Autodesk Inventor part; units mm, degrees
(part 2 of 2)
sketch "スケッチ13" plane through (0, 0, -5) normal (0, 0, -1) x (-1, 0, 0)
  arc A0 (74.152214, 49.824752) -> (76.907606, 48.647957) centre (77.811872, 54.579424) ccw
  arc A1 (74.152214, 49.824752) -> (72.542276, 49.029257) centre (73.542271, 49.032306) ccw
  arc A2 (70.331118, 43.4429) -> (72.542276, 49.029257) centre (64.442314, 49.004554) ccw
  arc A3 (70.331118, 43.4429) -> (70.457765, 41.956551) centre (71.058131, 42.756277) ccw
  line L0 (70.457765, 41.956551) -> (77.631528, 36.571106)
  arc A4 (77.631528, 36.571106) -> (79.072459, 36.829123) centre (78.231893, 37.370832) ccw
  arc A5 (80.094406, 38.031727) -> (79.072459, 36.829123) centre (84.115857, 33.578871) ccw
  arc A6 (80.094406, 38.031727) -> (80.381942, 39.061377) centre (79.424164, 38.77387) ccw
  line L1 (80.381942, 39.061377) -> (77.714673, 47.946886)
  arc A7 (77.714673, 47.946886) -> (76.907606, 48.647957) centre (76.756895, 47.659379) ccw
  arc A8 (137.500173, 2.708082) -> (138.19969, 1.899667) centre (138.489039, 2.856891) ccw
  arc A9 (142.031716, -1.608501) -> (138.19969, 1.899667) centre (136.463592, -3.843674) ccw
  arc A10 (142.031716, -1.608501) -> (143.581885, -2.018871) centre (142.959736, -1.235972) ccw
  line L2 (143.581885, -2.018871) -> (146.594315, 0.375026)
  arc A11 (146.594315, 0.375026) -> (146.254963, 2.117105) centre (145.972167, 1.157925) ccw
  arc A12 (142.242708, 6.02639) -> (146.254963, 2.117105) centre (147.951739, 7.872185) ccw
  arc A13 (142.242708, 6.02639) -> (141.421042, 6.710292) centre (141.291203, 5.718757) ccw
  line L3 (141.421042, 6.710292) -> (138.123227, 7.142135)
  arc A14 (138.123227, 7.142135) -> (137.004522, 6.001791) centre (137.993388, 6.1506) ccw
  line L4 (137.004522, 6.001791) -> (137.500173, 2.708082)
  arc A15 (136.03468, 16.286601) -> (138.023268, 18.525143) centre (132.685182, 21.264639) ccw
  arc A16 (136.03468, 16.286601) -> (135.604064, 15.308119) centre (136.59293, 15.456928) ccw
  line L5 (135.604064, 15.308119) -> (136.075602, 12.174654)
  arc A17 (136.075602, 12.174654) -> (136.934628, 11.331928) centre (137.064468, 12.323463) ccw
  line L6 (136.934628, 11.331928) -> (141.9404, 10.676432)
  arc A18 (141.9404, 10.676432) -> (142.910454, 11.125713) centre (142.07024, 11.667967) ccw
  arc A19 (145.546046, 13.368787) -> (142.910454, 11.125713) centre (147.951739, 7.872185) ccw
  arc A20 (145.546046, 13.368787) -> (145.664062, 15.139683) centre (145.145097, 14.284888) ccw
  line L7 (145.664062, 15.139683) -> (139.431914, 18.923356)
  arc A21 (139.431914, 18.923356) -> (138.023268, 18.525143) centre (138.912949, 18.068561) ccw
  arc A22 (100.355268, 41.394209) -> (100.058689, 42.827701) centre (99.539724, 41.972905) ccw
  line L8 (100.058689, 42.827701) -> (84.558604, 52.238141)
  arc A23 (84.558604, 52.238141) -> (83.149958, 51.839928) centre (84.039639, 51.383346) ccw
  arc A24 (81.833323, 50.126568) -> (83.149958, 51.839928) centre (77.811872, 54.579424) ccw
  arc A25 (81.833323, 50.126568) -> (81.545787, 49.096917) centre (82.503565, 49.384425) ccw
  line L9 (81.545787, 49.096917) -> (84.213055, 40.211408)
  arc A26 (84.213055, 40.211408) -> (85.020123, 39.510338) centre (85.170834, 40.498916) ccw
  arc A27 (88.908264, 37.188973) -> (85.020123, 39.510338) centre (84.115857, 33.578871) ccw
  arc A28 (88.908264, 37.188973) -> (89.908309, 36.81113) centre (89.706998, 37.790657) ccw
  line L10 (89.908309, 36.81113) -> (98.650829, 38.607882)
  arc A29 (98.650829, 38.607882) -> (99.420805, 39.349498) centre (98.449518, 39.587409) ccw
  arc A30 (100.355268, 41.394209) -> (99.420805, 39.349498) centre (105.248527, 37.922031) ccw
  arc A31 (70.160292, 54.741689) -> (71.858452, 55.325612) centre (70.866216, 55.449977) ccw
  arc A32 (72.918613, 58.051601) -> (71.858452, 55.325612) centre (77.811872, 54.579424) ccw
  arc A33 (72.918613, 58.051601) -> (72.622035, 59.485093) centre (72.10307, 58.630298) ccw
  line L11 (72.622035, 59.485093) -> (69.229438, 61.544813)
  arc A34 (69.229438, 61.544813) -> (67.802662, 61.109398) centre (68.710473, 60.690017) ccw
  arc A35 (66.414464, 59.026602) -> (67.802662, 61.109398) centre (60.449397, 64.50638) ccw
  arc A36 (66.414464, 59.026602) -> (66.550527, 57.55036) centre (67.150892, 58.350086) ccw
  line L12 (66.550527, 57.55036) -> (69.305274, 55.482332)
  arc A37 (70.160292, 54.741689) -> (69.305274, 55.482332) centre (64.442314, 49.004554) ccw
  arc A38 (127.791923, 24.736817) -> (126.690727, 21.522538) centre (132.685182, 21.264639) ccw
  arc A39 (127.791923, 24.736817) -> (127.495344, 26.170308) centre (126.976379, 25.315513) ccw
  line L13 (127.495344, 26.170308) -> (111.995259, 35.580749)
  arc A40 (111.995259, 35.580749) -> (110.586613, 35.182536) centre (111.476294, 34.725953) ccw
  arc A41 (109.14609, 33.360343) -> (110.586613, 35.182536) centre (105.248527, 37.922031) ccw
  arc A42 (109.14609, 33.360343) -> (108.830366, 32.338983) centre (109.795684, 32.600062) ccw
  line L14 (108.830366, 32.338983) -> (112.38569, 19.19344)
  arc A43 (112.38569, 19.19344) -> (113.173186, 18.470456) centre (113.351007, 19.454519) ccw
  arc A44 (116.098395, 17.045236) -> (113.173186, 18.470456) centre (112.106259, 12.566079) ccw
  arc A45 (116.098395, 17.045236) -> (117.15309, 16.870668) centre (116.763751, 17.791763) ccw
  line L15 (117.15309, 16.870668) -> (126.080991, 20.644427)
  arc A46 (126.080991, 20.644427) -> (126.690727, 21.522538) centre (125.691651, 21.565521) ccw
  line L16 (123.324226, 13.114183) -> (130.745103, 12.142434)
  arc A47 (130.745103, 12.142434) -> (131.863809, 13.282778) centre (130.874943, 13.133969) ccw
  line L17 (131.863809, 13.282778) -> (131.6486, 14.712884)
  arc A48 (131.6486, 14.712884) -> (130.949084, 15.521298) centre (130.659734, 14.564075) ccw
  arc A49 (128.693046, 16.785482) -> (130.949084, 15.521298) centre (132.685182, 21.264639) ccw
  arc A50 (128.693046, 16.785482) -> (127.63835, 16.96005) centre (128.02769, 16.038956) ccw
  line L18 (127.63835, 16.96005) -> (123.064726, 15.026812)
  arc A51 (123.064726, 15.026812) -> (123.324226, 13.114183) centre (123.454066, 14.105718) ccw
  arc A52 (88.644656, 29.643139) -> (88.79909, 28.187458) centre (89.399456, 28.987184) ccw
  line L19 (88.79909, 28.187458) -> (105.621929, 15.558314)
  arc A53 (105.621929, 15.558314) -> (107.062861, 15.816331) centre (106.222295, 16.35804) ccw
  arc A54 (108.208695, 17.127767) -> (107.062861, 15.816331) centre (112.106259, 12.566079) ccw
  arc A55 (108.208695, 17.127767) -> (108.524419, 18.149127) centre (107.559102, 17.888049) ccw
  line L20 (108.524419, 18.149127) -> (104.969096, 31.29467)
  arc A56 (104.969096, 31.29467) -> (104.181599, 32.017655) centre (104.003778, 31.033592) ccw
  arc A57 (100.45612, 34.311929) -> (104.181599, 32.017655) centre (105.248527, 37.922031) ccw
  arc A58 (100.45612, 34.311929) -> (99.456074, 34.689773) centre (99.657386, 33.710245) ccw
  line L21 (99.456074, 34.689773) -> (90.713554, 32.89302)
  arc A59 (90.713554, 32.89302) -> (89.943579, 32.151404) centre (90.914866, 31.913493) ccw
  arc A60 (88.644656, 29.643139) -> (89.943579, 32.151404) centre (84.115857, 33.578871) ccw
  arc A61 (133.114093, 1.134364) -> (133.54471, 2.112846) centre (132.555844, 1.964037) ccw
  line L22 (133.54471, 2.112846) -> (132.792729, 7.109914)
  arc A62 (132.792729, 7.109914) -> (131.933702, 7.95264) centre (131.803863, 6.961105) ccw
  line L23 (131.933702, 7.95264) -> (118.117598, 9.761832)
  arc A63 (118.117598, 9.761832) -> (117.147544, 9.312551) centre (117.987758, 8.770297) ccw
  arc A64 (116.635058, 8.630348) -> (117.147544, 9.312551) centre (112.106259, 12.566079) ccw
  arc A65 (116.635058, 8.630348) -> (116.789492, 7.174667) centre (117.389857, 7.974392) ccw
  line L24 (116.789492, 7.174667) -> (129.297772, -2.215477)
  arc A66 (129.297772, -2.215477) -> (130.83606, -1.762597) centre (129.898137, -1.415751) ccw
  arc A67 (133.114093, 1.134364) -> (130.83606, -1.762597) centre (136.463592, -3.843674) ccw
  circle A68 centre (105.248527, 37.922031) radius 3
  circle A69 centre (132.685182, 21.264639) radius 3
  circle A70 centre (77.811872, 54.579424) radius 3
  circle A71 centre (112.106259, 12.566079) radius 3
  circle A72 centre (84.115857, 33.578871) radius 3
  circle A73 centre (136.463592, -3.843674) radius 3
  circle A74 centre (147.951739, 7.872185) radius 3
  line L25 (46.496021, 71.105048) -> (58.588264, 62.02723)
  arc A75 (58.588264, 62.02723) -> (62.310529, 66.98553) centre (60.449397, 64.50638) ccw
  line L26 (62.310529, 66.98553) -> (56.416161, 71.410515)
  line L27 (56.416161, 71.410515) -> (60.233181, 71.528052)
  arc A76 (64.095126, 70.511318) -> (60.233181, 71.528052) centre (60.449397, 64.50638) ccw
  line L28 (64.095126, 70.511318) -> (136.058454, 26.82081)
  arc A77 (136.850058, 26.255011) -> (136.058454, 26.82081) centre (132.685182, 21.264639) ccw
  line L29 (136.850058, 26.255011) -> (152.436991, 13.246431)
  arc A78 (153.239213, 3.284961) -> (152.436991, 13.246431) centre (147.951739, 7.872185) ccw
  line L30 (153.239213, 3.284961) -> (142.506418, -9.086216)
  arc A79 (131.660668, -10.24148) -> (142.506418, -9.086216) centre (136.463592, -3.843674) ccw
  line L31 (131.660668, -10.24148) -> (40.231602, 58.395617)
  arc A80 (37.546552, 65.319255) -> (40.231602, 58.395617) centre (44.44917, 64.013691) ccw
  line L32 (37.546552, 65.319255) -> (62.581181, 46.525404)
  arc A81 (62.581181, 46.525404) -> (66.303447, 51.483704) centre (64.442314, 49.004554) ccw
  line L33 (66.303447, 51.483704) -> (41.268818, 70.277554)
  arc A82 (44.232954, 71.035362) -> (41.268818, 70.277554) centre (44.44917, 64.013691) ccw
  line L34 (44.232954, 71.035362) -> (46.496021, 71.105048)
  circle A83 centre (147.951739, 7.872185) radius 7
  point P0 (0, 0)
  point P1 (146.087496, 14.619377)
  point P2 (141.559999, 10.726245)
  point P3 (141.040641, 6.760105)
  point P4 (146.949096, 0.944364)
  dimension "d69" = 4
  constraints: 1 centre point, 1 coincident
  measures "d69" radial gap between concentric circles of A74 A83
extrude "押し出し11" add sketch "スケッチ13" against normal blind 5 contours L3 A13 A12 A11 A83 | A83 A20 A19 A18 L6
fillet "フィレット2" radius 1 2 edges at (-146.9491, 0.9444, -3) (-146.0875, 14.6194, -3)
fillet "フィレット3" radius 1 2 edges at (-141.0406, 6.7601, -3) (-141.56, 10.7262, -3)
sketch "スケッチ14" plane through (0, 0, -5) normal (0, 0, -1) x (-1, 0, 0)
  arc A0 (74.152214, 49.824752) -> (76.907606, 48.647957) centre (77.811872, 54.579424) ccw
  arc A1 (74.152214, 49.824752) -> (72.542276, 49.029257) centre (73.542271, 49.032306) ccw
  arc A2 (70.331118, 43.4429) -> (72.542276, 49.029257) centre (64.442314, 49.004554) ccw
  arc A3 (70.331118, 43.4429) -> (70.457765, 41.956551) centre (71.058131, 42.756277) ccw
  line L0 (70.457765, 41.956551) -> (77.631528, 36.571106)
  arc A4 (77.631528, 36.571106) -> (79.072459, 36.829123) centre (78.231893, 37.370832) ccw
  arc A5 (80.094406, 38.031727) -> (79.072459, 36.829123) centre (84.115857, 33.578871) ccw
  arc A6 (80.094406, 38.031727) -> (80.381942, 39.061377) centre (79.424164, 38.77387) ccw
  line L1 (80.381942, 39.061377) -> (77.714673, 47.946886)
  arc A7 (77.714673, 47.946886) -> (76.907606, 48.647957) centre (76.756895, 47.659379) ccw
  arc A8 (137.500173, 2.708082) -> (138.19969, 1.899667) centre (138.489039, 2.856891) ccw
  arc A9 (142.031716, -1.608501) -> (138.19969, 1.899667) centre (136.463592, -3.843674) ccw
  arc A10 (142.031716, -1.608501) -> (143.581885, -2.018871) centre (142.959736, -1.235972) ccw
  line L2 (143.581885, -2.018871) -> (145.665299, -0.363238)
  arc A11 (145.665299, -0.363238) -> (145.406724, 1.351227) centre (145.043151, 0.419661) ccw
  arc A12 (141.176668, 6.111957) -> (145.406724, 1.351227) centre (147.951739, 7.872185) ccw
  arc A13 (141.176668, 6.111957) -> (140.33864, 6.852031) centre (140.2088, 5.860496) ccw
  line L3 (140.33864, 6.852031) -> (138.123227, 7.142135)
  arc A14 (138.123227, 7.142135) -> (137.004522, 6.001791) centre (137.993388, 6.1506) ccw
  line L4 (137.004522, 6.001791) -> (137.500173, 2.708082)
  arc A15 (136.03468, 16.286601) -> (138.023268, 18.525143) centre (132.685182, 21.264639) ccw
  arc A16 (136.03468, 16.286601) -> (135.604064, 15.308119) centre (136.59293, 15.456928) ccw
  line L5 (135.604064, 15.308119) -> (136.075602, 12.174654)
  arc A17 (136.075602, 12.174654) -> (136.934628, 11.331928) centre (137.064468, 12.323463) ccw
  line L6 (136.934628, 11.331928) -> (140.857998, 10.818171)
  arc A18 (140.857998, 10.818171) -> (141.858325, 11.317516) centre (140.987838, 11.809706) ccw
  arc A19 (144.608388, 14.022144) -> (141.858325, 11.317516) centre (147.951739, 7.872185) ccw
  arc A20 (144.608388, 14.022144) -> (144.649731, 15.755505) centre (144.130766, 14.90071) ccw
  line L7 (144.649731, 15.755505) -> (139.431914, 18.923356)
  arc A21 (139.431914, 18.923356) -> (138.023268, 18.525143) centre (138.912949, 18.068561) ccw
  arc A22 (100.355268, 41.394209) -> (100.058689, 42.827701) centre (99.539724, 41.972905) ccw
  line L8 (100.058689, 42.827701) -> (84.558604, 52.238141)
  arc A23 (84.558604, 52.238141) -> (83.149958, 51.839928) centre (84.039639, 51.383346) ccw
  arc A24 (81.833323, 50.126568) -> (83.149958, 51.839928) centre (77.811872, 54.579424) ccw
  arc A25 (81.833323, 50.126568) -> (81.545787, 49.096917) centre (82.503565, 49.384425) ccw
  line L9 (81.545787, 49.096917) -> (84.213055, 40.211408)
  arc A26 (84.213055, 40.211408) -> (85.020123, 39.510338) centre (85.170834, 40.498916) ccw
  arc A27 (88.908264, 37.188973) -> (85.020123, 39.510338) centre (84.115857, 33.578871) ccw
  arc A28 (88.908264, 37.188973) -> (89.908309, 36.81113) centre (89.706998, 37.790657) ccw
  line L10 (89.908309, 36.81113) -> (98.650829, 38.607882)
  arc A29 (98.650829, 38.607882) -> (99.420805, 39.349498) centre (98.449518, 39.587409) ccw
  arc A30 (100.355268, 41.394209) -> (99.420805, 39.349498) centre (105.248527, 37.922031) ccw
  arc A31 (70.160292, 54.741689) -> (71.858452, 55.325612) centre (70.866216, 55.449977) ccw
  arc A32 (72.918613, 58.051601) -> (71.858452, 55.325612) centre (77.811872, 54.579424) ccw
  arc A33 (72.918613, 58.051601) -> (72.622035, 59.485093) centre (72.10307, 58.630298) ccw
  line L11 (72.622035, 59.485093) -> (69.229438, 61.544813)
  arc A34 (69.229438, 61.544813) -> (67.802662, 61.109398) centre (68.710473, 60.690017) ccw
  arc A35 (66.414464, 59.026602) -> (67.802662, 61.109398) centre (60.449397, 64.50638) ccw
  arc A36 (66.414464, 59.026602) -> (66.550527, 57.55036) centre (67.150892, 58.350086) ccw
  line L12 (66.550527, 57.55036) -> (69.305274, 55.482332)
  arc A37 (70.160292, 54.741689) -> (69.305274, 55.482332) centre (64.442314, 49.004554) ccw
  arc A38 (127.791923, 24.736817) -> (126.690727, 21.522538) centre (132.685182, 21.264639) ccw
  arc A39 (127.791923, 24.736817) -> (127.495344, 26.170308) centre (126.976379, 25.315513) ccw
  line L13 (127.495344, 26.170308) -> (111.995259, 35.580749)
  arc A40 (111.995259, 35.580749) -> (110.586613, 35.182536) centre (111.476294, 34.725953) ccw
  arc A41 (109.14609, 33.360343) -> (110.586613, 35.182536) centre (105.248527, 37.922031) ccw
  arc A42 (109.14609, 33.360343) -> (108.830366, 32.338983) centre (109.795684, 32.600062) ccw
  line L14 (108.830366, 32.338983) -> (112.38569, 19.19344)
  arc A43 (112.38569, 19.19344) -> (113.173186, 18.470456) centre (113.351007, 19.454519) ccw
  arc A44 (116.098395, 17.045236) -> (113.173186, 18.470456) centre (112.106259, 12.566079) ccw
  arc A45 (116.098395, 17.045236) -> (117.15309, 16.870668) centre (116.763751, 17.791763) ccw
  line L15 (117.15309, 16.870668) -> (126.080991, 20.644427)
  arc A46 (126.080991, 20.644427) -> (126.690727, 21.522538) centre (125.691651, 21.565521) ccw
  line L16 (123.324226, 13.114183) -> (130.745103, 12.142434)
  arc A47 (130.745103, 12.142434) -> (131.863809, 13.282778) centre (130.874943, 13.133969) ccw
  line L17 (131.863809, 13.282778) -> (131.6486, 14.712884)
  arc A48 (131.6486, 14.712884) -> (130.949084, 15.521298) centre (130.659734, 14.564075) ccw
  arc A49 (128.693046, 16.785482) -> (130.949084, 15.521298) centre (132.685182, 21.264639) ccw
  arc A50 (128.693046, 16.785482) -> (127.63835, 16.96005) centre (128.02769, 16.038956) ccw
  line L18 (127.63835, 16.96005) -> (123.064726, 15.026812)
  arc A51 (123.064726, 15.026812) -> (123.324226, 13.114183) centre (123.454066, 14.105718) ccw
  arc A52 (88.644656, 29.643139) -> (88.79909, 28.187458) centre (89.399456, 28.987184) ccw
  line L19 (88.79909, 28.187458) -> (105.621929, 15.558314)
  arc A53 (105.621929, 15.558314) -> (107.062861, 15.816331) centre (106.222295, 16.35804) ccw
  arc A54 (108.208695, 17.127767) -> (107.062861, 15.816331) centre (112.106259, 12.566079) ccw
  arc A55 (108.208695, 17.127767) -> (108.524419, 18.149127) centre (107.559102, 17.888049) ccw
  line L20 (108.524419, 18.149127) -> (104.969096, 31.29467)
  arc A56 (104.969096, 31.29467) -> (104.181599, 32.017655) centre (104.003778, 31.033592) ccw
  arc A57 (100.45612, 34.311929) -> (104.181599, 32.017655) centre (105.248527, 37.922031) ccw
  arc A58 (100.45612, 34.311929) -> (99.456074, 34.689773) centre (99.657386, 33.710245) ccw
  line L21 (99.456074, 34.689773) -> (90.713554, 32.89302)
  arc A59 (90.713554, 32.89302) -> (89.943579, 32.151404) centre (90.914866, 31.913493) ccw
  arc A60 (88.644656, 29.643139) -> (89.943579, 32.151404) centre (84.115857, 33.578871) ccw
  arc A61 (133.114093, 1.134364) -> (133.54471, 2.112846) centre (132.555844, 1.964037) ccw
  line L22 (133.54471, 2.112846) -> (132.792729, 7.109914)
  arc A62 (132.792729, 7.109914) -> (131.933702, 7.95264) centre (131.803863, 6.961105) ccw
  line L23 (131.933702, 7.95264) -> (118.117598, 9.761832)
  arc A63 (118.117598, 9.761832) -> (117.147544, 9.312551) centre (117.987758, 8.770297) ccw
  arc A64 (116.635058, 8.630348) -> (117.147544, 9.312551) centre (112.106259, 12.566079) ccw
  arc A65 (116.635058, 8.630348) -> (116.789492, 7.174667) centre (117.389857, 7.974392) ccw
  line L24 (116.789492, 7.174667) -> (129.297772, -2.215477)
  arc A66 (129.297772, -2.215477) -> (130.83606, -1.762597) centre (129.898137, -1.415751) ccw
  arc A67 (133.114093, 1.134364) -> (130.83606, -1.762597) centre (136.463592, -3.843674) ccw
  circle A68 centre (105.248527, 37.922031) radius 3
  circle A69 centre (132.685182, 21.264639) radius 3
  circle A70 centre (77.811872, 54.579424) radius 3
  circle A71 centre (112.106259, 12.566079) radius 3
  circle A72 centre (84.115857, 33.578871) radius 3
  circle A73 centre (136.463592, -3.843674) radius 3
  circle A74 centre (147.951739, 7.872185) radius 3
  line L25 (46.496021, 71.105048) -> (58.588264, 62.02723)
  arc A75 (58.588264, 62.02723) -> (62.310529, 66.98553) centre (60.449397, 64.50638) ccw
  line L26 (62.310529, 66.98553) -> (56.416161, 71.410515)
  line L27 (56.416161, 71.410515) -> (60.233181, 71.528052)
  arc A76 (64.095126, 70.511318) -> (60.233181, 71.528052) centre (60.449397, 64.50638) ccw
  line L28 (64.095126, 70.511318) -> (136.058454, 26.82081)
  arc A77 (136.850058, 26.255011) -> (136.058454, 26.82081) centre (132.685182, 21.264639) ccw
  line L29 (136.850058, 26.255011) -> (152.436991, 13.246431)
  arc A78 (153.239213, 3.284961) -> (152.436991, 13.246431) centre (147.951739, 7.872185) ccw
  line L30 (153.239213, 3.284961) -> (142.506418, -9.086216)
  arc A79 (131.660668, -10.24148) -> (142.506418, -9.086216) centre (136.463592, -3.843674) ccw
  line L31 (131.660668, -10.24148) -> (40.231602, 58.395617)
  arc A80 (37.546552, 65.319255) -> (40.231602, 58.395617) centre (44.44917, 64.013691) ccw
  line L32 (37.546552, 65.319255) -> (62.581181, 46.525404)
  arc A81 (62.581181, 46.525404) -> (66.303447, 51.483704) centre (64.442314, 49.004554) ccw
  line L33 (66.303447, 51.483704) -> (41.268818, 70.277554)
  arc A82 (44.232954, 71.035362) -> (41.268818, 70.277554) centre (44.44917, 64.013691) ccw
  line L34 (44.232954, 71.035362) -> (46.496021, 71.105048)
  point P0 (0, 0)
sketch "スケッチ15" plane through (0, 0, -5) normal (0, 0, -1) x (-1, 0, 0)
  arc A0 (131.660668, -10.24148) -> (142.506418, -9.086216) centre (136.463592, -3.843674) ccw
  line L0 (131.660668, -10.24148) -> (40.231602, 58.395617)
  arc A1 (44.232954, 71.035362) -> (40.231602, 58.395617) centre (44.44917, 64.013691) ccw
  line L1 (44.232954, 71.035362) -> (60.233181, 71.528052)
  arc A2 (64.095126, 70.511318) -> (60.233181, 71.528052) centre (60.449397, 64.50638) ccw
  line L2 (64.095126, 70.511318) -> (136.058454, 26.82081)
  arc A3 (136.850058, 26.255011) -> (136.058454, 26.82081) centre (132.685182, 21.264639) ccw
  line L3 (136.850058, 26.255011) -> (152.436991, 13.246431)
  arc A4 (153.239213, 3.284961) -> (152.436991, 13.246431) centre (147.951739, 7.872185) ccw
  line L4 (153.239213, 3.284961) -> (142.506418, -9.086216)
  circle A5 centre (132.685182, 21.264639) radius 3
  circle A6 centre (147.951739, 7.872185) radius 3
  circle A7 centre (136.463592, -3.843674) radius 3
  circle A8 centre (84.115857, 33.578871) radius 1.5
  circle A9 centre (105.248527, 37.922031) radius 1.5
  circle A10 centre (77.811872, 54.579424) radius 1.5
  circle A11 centre (112.106259, 12.566079) radius 1.5
  circle A12 centre (60.449397, 64.50638) radius 1.5
  circle A13 centre (64.442314, 49.004554) radius 1.5
  circle A14 centre (44.44917, 64.013691) radius 1.5
  line L5 (149.23324, 9.407684) -> (133.646307, 22.416263)
  arc A15 (133.646307, 22.416263) -> (133.463629, 22.546832) centre (132.685182, 21.264639) ccw
  line L6 (133.463629, 22.546832) -> (61.500301, 66.237341)
  arc A16 (61.500301, 66.237341) -> (60.387071, 66.53042) centre (60.449397, 64.50638) ccw
  line L7 (60.387071, 66.53042) -> (44.386844, 66.037731)
  arc A17 (44.386844, 66.037731) -> (43.23343, 62.394246) centre (44.44917, 64.013691) ccw
  line L8 (43.23343, 62.394246) -> (134.662496, -6.242851)
  arc A18 (134.662496, -6.242851) -> (138.729652, -5.809627) centre (136.463592, -3.843674) ccw
  line L9 (138.729652, -5.809627) -> (149.462446, 6.561549)
  arc A19 (149.462446, 6.561549) -> (149.23324, 9.407684) centre (147.951739, 7.872185) ccw
  arc A20 (74.152214, 49.824752) -> (76.907606, 48.647957) centre (77.811872, 54.579424) ccw
  arc A21 (74.152214, 49.824752) -> (72.542276, 49.029257) centre (73.542271, 49.032306) ccw
  arc A22 (70.331118, 43.4429) -> (72.542276, 49.029257) centre (64.442314, 49.004554) ccw
  arc A23 (70.331118, 43.4429) -> (70.457765, 41.956551) centre (71.058131, 42.756277) ccw
  line L10 (70.457765, 41.956551) -> (77.631528, 36.571106)
  arc A24 (77.631528, 36.571106) -> (79.072459, 36.829123) centre (78.231893, 37.370832) ccw
  arc A25 (80.094406, 38.031727) -> (79.072459, 36.829123) centre (84.115857, 33.578871) ccw
  arc A26 (80.094406, 38.031727) -> (80.381942, 39.061377) centre (79.424164, 38.77387) ccw
  line L11 (80.381942, 39.061377) -> (77.714673, 47.946886)
  arc A27 (77.714673, 47.946886) -> (76.907606, 48.647957) centre (76.756895, 47.659379) ccw
  arc A28 (137.500173, 2.708082) -> (138.19969, 1.899667) centre (138.489039, 2.856891) ccw
  arc A29 (142.031716, -1.608501) -> (138.19969, 1.899667) centre (136.463592, -3.843674) ccw
  arc A30 (142.031716, -1.608501) -> (143.581885, -2.018871) centre (142.959736, -1.235972) ccw
  line L12 (143.581885, -2.018871) -> (145.665299, -0.363238)
  arc A31 (145.665299, -0.363238) -> (145.406724, 1.351227) centre (145.043151, 0.419661) ccw
  arc A32 (141.176668, 6.111957) -> (145.406724, 1.351227) centre (147.951739, 7.872185) ccw
  arc A33 (141.176668, 6.111957) -> (140.33864, 6.852031) centre (140.2088, 5.860496) ccw
  line L13 (140.33864, 6.852031) -> (138.123227, 7.142135)
  arc A34 (138.123227, 7.142135) -> (137.004522, 6.001791) centre (137.993388, 6.1506) ccw
  line L14 (137.004522, 6.001791) -> (137.500173, 2.708082)
  arc A35 (136.03468, 16.286601) -> (138.023268, 18.525143) centre (132.685182, 21.264639) ccw
  arc A36 (136.03468, 16.286601) -> (135.604064, 15.308119) centre (136.59293, 15.456928) ccw
  line L15 (135.604064, 15.308119) -> (136.075602, 12.174654)
  arc A37 (136.075602, 12.174654) -> (136.934628, 11.331928) centre (137.064468, 12.323463) ccw
  line L16 (136.934628, 11.331928) -> (140.857998, 10.818171)
  arc A38 (140.857998, 10.818171) -> (141.858325, 11.317516) centre (140.987838, 11.809706) ccw
  arc A39 (144.608388, 14.022144) -> (141.858325, 11.317516) centre (147.951739, 7.872185) ccw
  arc A40 (144.608388, 14.022144) -> (144.649731, 15.755505) centre (144.130766, 14.90071) ccw
  line L17 (144.649731, 15.755505) -> (139.431914, 18.923356)
  arc A41 (139.431914, 18.923356) -> (138.023268, 18.525143) centre (138.912949, 18.068561) ccw
  arc A42 (100.355268, 41.394209) -> (100.058689, 42.827701) centre (99.539724, 41.972905) ccw
  line L18 (100.058689, 42.827701) -> (84.558604, 52.238141)
  arc A43 (84.558604, 52.238141) -> (83.149958, 51.839928) centre (84.039639, 51.383346) ccw
  arc A44 (81.833323, 50.126568) -> (83.149958, 51.839928) centre (77.811872, 54.579424) ccw
  arc A45 (81.833323, 50.126568) -> (81.545787, 49.096917) centre (82.503565, 49.384425) ccw
  line L19 (81.545787, 49.096917) -> (84.213055, 40.211408)
  arc A46 (84.213055, 40.211408) -> (85.020123, 39.510338) centre (85.170834, 40.498916) ccw
  arc A47 (88.908264, 37.188973) -> (85.020123, 39.510338) centre (84.115857, 33.578871) ccw
  arc A48 (88.908264, 37.188973) -> (89.908309, 36.81113) centre (89.706998, 37.790657) ccw
  line L20 (89.908309, 36.81113) -> (98.650829, 38.607882)
  arc A49 (98.650829, 38.607882) -> (99.420805, 39.349498) centre (98.449518, 39.587409) ccw
  arc A50 (100.355268, 41.394209) -> (99.420805, 39.349498) centre (105.248527, 37.922031) ccw
  arc A51 (70.160292, 54.741689) -> (71.858452, 55.325612) centre (70.866216, 55.449977) ccw
  arc A52 (72.918613, 58.051601) -> (71.858452, 55.325612) centre (77.811872, 54.579424) ccw
  arc A53 (72.918613, 58.051601) -> (72.622035, 59.485093) centre (72.10307, 58.630298) ccw
  line L21 (72.622035, 59.485093) -> (69.229438, 61.544813)
  arc A54 (69.229438, 61.544813) -> (67.802662, 61.109398) centre (68.710473, 60.690017) ccw
  arc A55 (66.414464, 59.026602) -> (67.802662, 61.109398) centre (60.449397, 64.50638) ccw
  arc A56 (66.414464, 59.026602) -> (66.550527, 57.55036) centre (67.150892, 58.350086) ccw
  line L22 (66.550527, 57.55036) -> (69.305274, 55.482332)
  arc A57 (70.160292, 54.741689) -> (69.305274, 55.482332) centre (64.442314, 49.004554) ccw
  arc A58 (127.791923, 24.736817) -> (126.690727, 21.522538) centre (132.685182, 21.264639) ccw
  arc A59 (127.791923, 24.736817) -> (127.495344, 26.170308) centre (126.976379, 25.315513) ccw
  line L23 (127.495344, 26.170308) -> (111.995259, 35.580749)
  arc A60 (111.995259, 35.580749) -> (110.586613, 35.182536) centre (111.476294, 34.725953) ccw
  arc A61 (109.14609, 33.360343) -> (110.586613, 35.182536) centre (105.248527, 37.922031) ccw
  arc A62 (109.14609, 33.360343) -> (108.830366, 32.338983) centre (109.795684, 32.600062) ccw
  line L24 (108.830366, 32.338983) -> (112.38569, 19.19344)
  arc A63 (112.38569, 19.19344) -> (113.173186, 18.470456) centre (113.351007, 19.454519) ccw
  arc A64 (116.098395, 17.045236) -> (113.173186, 18.470456) centre (112.106259, 12.566079) ccw
  arc A65 (116.098395, 17.045236) -> (117.15309, 16.870668) centre (116.763751, 17.791763) ccw
  line L25 (117.15309, 16.870668) -> (126.080991, 20.644427)
  arc A66 (126.080991, 20.644427) -> (126.690727, 21.522538) centre (125.691651, 21.565521) ccw
  line L26 (123.324226, 13.114183) -> (130.745103, 12.142434)
  arc A67 (130.745103, 12.142434) -> (131.863809, 13.282778) centre (130.874943, 13.133969) ccw
  line L27 (131.863809, 13.282778) -> (131.6486, 14.712884)
  arc A68 (131.6486, 14.712884) -> (130.949084, 15.521298) centre (130.659734, 14.564075) ccw
  arc A69 (128.693046, 16.785482) -> (130.949084, 15.521298) centre (132.685182, 21.264639) ccw
  arc A70 (128.693046, 16.785482) -> (127.63835, 16.96005) centre (128.02769, 16.038956) ccw
  line L28 (127.63835, 16.96005) -> (123.064726, 15.026812)
  arc A71 (123.064726, 15.026812) -> (123.324226, 13.114183) centre (123.454066, 14.105718) ccw
  arc A72 (88.644656, 29.643139) -> (88.79909, 28.187458) centre (89.399456, 28.987184) ccw
  line L29 (88.79909, 28.187458) -> (105.621929, 15.558314)
  arc A73 (105.621929, 15.558314) -> (107.062861, 15.816331) centre (106.222295, 16.35804) ccw
  arc A74 (108.208695, 17.127767) -> (107.062861, 15.816331) centre (112.106259, 12.566079) ccw
  arc A75 (108.208695, 17.127767) -> (108.524419, 18.149127) centre (107.559102, 17.888049) ccw
  line L30 (108.524419, 18.149127) -> (104.969096, 31.29467)
  arc A76 (104.969096, 31.29467) -> (104.181599, 32.017655) centre (104.003778, 31.033592) ccw
  arc A77 (100.45612, 34.311929) -> (104.181599, 32.017655) centre (105.248527, 37.922031) ccw
  arc A78 (100.45612, 34.311929) -> (99.456074, 34.689773) centre (99.657386, 33.710245) ccw
  line L31 (99.456074, 34.689773) -> (90.713554, 32.89302)
  arc A79 (90.713554, 32.89302) -> (89.943579, 32.151404) centre (90.914866, 31.913493) ccw
  arc A80 (88.644656, 29.643139) -> (89.943579, 32.151404) centre (84.115857, 33.578871) ccw
  arc A81 (133.114093, 1.134364) -> (133.54471, 2.112846) centre (132.555844, 1.964037) ccw
  line L32 (133.54471, 2.112846) -> (132.792729, 7.109914)
  arc A82 (132.792729, 7.109914) -> (131.933702, 7.95264) centre (131.803863, 6.961105) ccw
  line L33 (131.933702, 7.95264) -> (118.117598, 9.761832)
  arc A83 (118.117598, 9.761832) -> (117.147544, 9.312551) centre (117.987758, 8.770297) ccw
  arc A84 (116.635058, 8.630348) -> (117.147544, 9.312551) centre (112.106259, 12.566079) ccw
  arc A85 (116.635058, 8.630348) -> (116.789492, 7.174667) centre (117.389857, 7.974392) ccw
  line L34 (116.789492, 7.174667) -> (129.297772, -2.215477)
  arc A86 (129.297772, -2.215477) -> (130.83606, -1.762597) centre (129.898137, -1.415751) ccw
  arc A87 (133.114093, 1.134364) -> (130.83606, -1.762597) centre (136.463592, -3.843674) ccw
  circle A88 centre (105.248527, 37.922031) radius 3
  circle A89 centre (132.685182, 21.264639) radius 3
  circle A90 centre (77.811872, 54.579424) radius 3
  circle A91 centre (112.106259, 12.566079) radius 3
  circle A92 centre (84.115857, 33.578871) radius 3
  circle A93 centre (136.463592, -3.843674) radius 3
  circle A94 centre (147.951739, 7.872185) radius 3
  line L35 (46.496021, 71.105048) -> (58.588264, 62.02723)
  arc A95 (58.588264, 62.02723) -> (62.310529, 66.98553) centre (60.449397, 64.50638) ccw
  line L36 (62.310529, 66.98553) -> (56.416161, 71.410515)
  line L37 (56.416161, 71.410515) -> (60.233181, 71.528052)
  arc A96 (64.095126, 70.511318) -> (60.233181, 71.528052) centre (60.449397, 64.50638) ccw
  line L38 (64.095126, 70.511318) -> (136.058454, 26.82081)
  arc A97 (136.850058, 26.255011) -> (136.058454, 26.82081) centre (132.685182, 21.264639) ccw
  line L39 (136.850058, 26.255011) -> (152.436991, 13.246431)
  arc A98 (153.239213, 3.284961) -> (152.436991, 13.246431) centre (147.951739, 7.872185) ccw
  line L40 (153.239213, 3.284961) -> (142.506418, -9.086216)
  arc A99 (131.660668, -10.24148) -> (142.506418, -9.086216) centre (136.463592, -3.843674) ccw
  line L41 (131.660668, -10.24148) -> (40.231602, 58.395617)
  arc A100 (37.546552, 65.319255) -> (40.231602, 58.395617) centre (44.44917, 64.013691) ccw
  line L42 (37.546552, 65.319255) -> (62.581181, 46.525404)
  arc A101 (62.581181, 46.525404) -> (66.303447, 51.483704) centre (64.442314, 49.004554) ccw
  line L43 (66.303447, 51.483704) -> (41.268818, 70.277554)
  arc A102 (44.232954, 71.035362) -> (41.268818, 70.277554) centre (44.44917, 64.013691) ccw
  line L44 (44.232954, 71.035362) -> (46.496021, 71.105048)
  point P0 (0, 0)
  point P1 (145.066441, 1.494485)
  point P2 (142.167826, -1.846609)
  point P3 (138.122228, 18.680738)
  point P4 (144.08302, 13.705967)
  dimension "d74" = 5
  constraints: 10 end point, 10 point on circle, 5 centre point, 9 other
  measures "d74" distance between parallel lines of L3 L5
extrude "押し出し12" add sketch "スケッチ15" against normal blind 5 contours L9 A32 A31 L12 A30 | A41 L17 A40 A39 L5
fillet "フィレット4" radius 1 4 edges at (-142.1678, -1.8466, -3) (-145.0664, 1.4945, -3) (-144.083, 13.706, -3) (-138.1222, 18.6807, -3)
sketch "スケッチ16" plane through (0, 0, 0) normal (0, 0, 1) x (1, 0, 0)
  arc A0 (-142.506418, -9.086216) -> (-131.660668, -10.24148) centre (-136.463592, -3.843674) ccw
  line L0 (-142.506418, -9.086216) -> (-153.239213, 3.284961)
  arc A1 (-152.436991, 13.246431) -> (-153.239213, 3.284961) centre (-147.951739, 7.872185) ccw
  line L1 (-152.436991, 13.246431) -> (-136.850058, 26.255011)
  arc A2 (-136.058454, 26.82081) -> (-136.850058, 26.255011) centre (-132.685182, 21.264639) ccw
  line L2 (-136.058454, 26.82081) -> (-64.095126, 70.511318)
  arc A3 (-60.233181, 71.528052) -> (-64.095126, 70.511318) centre (-60.449397, 64.50638) ccw
  line L3 (-60.233181, 71.528052) -> (-56.416161, 71.410515)
  line L4 (-56.416161, 71.410515) -> (-62.310529, 66.98553)
  arc A4 (-62.310529, 66.98553) -> (-58.588264, 62.02723) centre (-60.449397, 64.50638) ccw
  line L5 (-58.588264, 62.02723) -> (-46.496021, 71.105048)
  line L6 (-46.496021, 71.105048) -> (-44.232954, 71.035362)
  arc A5 (-41.268818, 70.277554) -> (-44.232954, 71.035362) centre (-44.44917, 64.013691) ccw
  line L7 (-41.268818, 70.277554) -> (-66.303447, 51.483704)
  arc A6 (-66.303447, 51.483704) -> (-62.581181, 46.525404) centre (-64.442314, 49.004554) ccw
  line L8 (-62.581181, 46.525404) -> (-37.546552, 65.319255)
  arc A7 (-40.231602, 58.395617) -> (-37.546552, 65.319255) centre (-44.44917, 64.013691) ccw
  line L9 (-40.231602, 58.395617) -> (-131.660668, -10.24148)
  circle A8 centre (-147.951739, 7.872185) radius 3
  circle A9 centre (-136.463592, -3.843674) radius 3
  circle A10 centre (-84.115857, 33.578871) radius 3
  circle A11 centre (-112.106259, 12.566079) radius 3
  circle A12 centre (-77.811872, 54.579424) radius 3
  circle A13 centre (-132.685182, 21.264639) radius 3
  circle A14 centre (-105.248527, 37.922031) radius 3
  arc A15 (-133.54471, 2.112846) -> (-133.114093, 1.134364) centre (-132.555844, 1.964037) ccw
  arc A16 (-130.83606, -1.762597) -> (-133.114093, 1.134364) centre (-136.463592, -3.843674) ccw
  arc A17 (-130.83606, -1.762597) -> (-129.297772, -2.215477) centre (-129.898137, -1.415751) ccw
  line L10 (-129.297772, -2.215477) -> (-116.789492, 7.174667)
  arc A18 (-116.789492, 7.174667) -> (-116.635058, 8.630348) centre (-117.389857, 7.974392) ccw
  arc A19 (-117.147544, 9.312551) -> (-116.635058, 8.630348) centre (-112.106259, 12.566079) ccw
  arc A20 (-117.147544, 9.312551) -> (-118.117598, 9.761832) centre (-117.987758, 8.770297) ccw
  line L11 (-118.117598, 9.761832) -> (-131.933702, 7.95264)
  arc A21 (-131.933702, 7.95264) -> (-132.792729, 7.109914) centre (-131.803863, 6.961105) ccw
  line L12 (-132.792729, 7.109914) -> (-133.54471, 2.112846)
  arc A22 (-88.79909, 28.187458) -> (-88.644656, 29.643139) centre (-89.399456, 28.987184) ccw
  arc A23 (-89.943579, 32.151404) -> (-88.644656, 29.643139) centre (-84.115857, 33.578871) ccw
  arc A24 (-89.943579, 32.151404) -> (-90.713554, 32.89302) centre (-90.914866, 31.913493) ccw
  line L13 (-90.713554, 32.89302) -> (-99.456074, 34.689773)
  arc A25 (-99.456074, 34.689773) -> (-100.45612, 34.311929) centre (-99.657386, 33.710245) ccw
  arc A26 (-104.181599, 32.017655) -> (-100.45612, 34.311929) centre (-105.248527, 37.922031) ccw
  arc A27 (-104.181599, 32.017655) -> (-104.969096, 31.29467) centre (-104.003778, 31.033592) ccw
  line L14 (-104.969096, 31.29467) -> (-108.524419, 18.149127)
  arc A28 (-108.524419, 18.149127) -> (-108.208695, 17.127767) centre (-107.559102, 17.888049) ccw
  arc A29 (-107.062861, 15.816331) -> (-108.208695, 17.127767) centre (-112.106259, 12.566079) ccw
  arc A30 (-107.062861, 15.816331) -> (-105.621929, 15.558314) centre (-106.222295, 16.35804) ccw
  line L15 (-105.621929, 15.558314) -> (-88.79909, 28.187458)
  line L16 (-130.745103, 12.142434) -> (-123.324226, 13.114183)
  arc A31 (-123.324226, 13.114183) -> (-123.064726, 15.026812) centre (-123.454066, 14.105718) ccw
  line L17 (-123.064726, 15.026812) -> (-127.63835, 16.96005)
  arc A32 (-127.63835, 16.96005) -> (-128.693046, 16.785482) centre (-128.02769, 16.038956) ccw
  arc A33 (-130.949084, 15.521298) -> (-128.693046, 16.785482) centre (-132.685182, 21.264639) ccw
  arc A34 (-130.949084, 15.521298) -> (-131.6486, 14.712884) centre (-130.659734, 14.564075) ccw
  line L18 (-131.6486, 14.712884) -> (-131.863809, 13.282778)
  arc A35 (-131.863809, 13.282778) -> (-130.745103, 12.142434) centre (-130.874943, 13.133969) ccw
  arc A36 (-126.690727, 21.522538) -> (-127.791923, 24.736817) centre (-132.685182, 21.264639) ccw
  arc A37 (-126.690727, 21.522538) -> (-126.080991, 20.644427) centre (-125.691651, 21.565521) ccw
  line L19 (-126.080991, 20.644427) -> (-117.15309, 16.870668)
  arc A38 (-117.15309, 16.870668) -> (-116.098395, 17.045236) centre (-116.763751, 17.791763) ccw
  arc A39 (-113.173186, 18.470456) -> (-116.098395, 17.045236) centre (-112.106259, 12.566079) ccw
  arc A40 (-113.173186, 18.470456) -> (-112.38569, 19.19344) centre (-113.351007, 19.454519) ccw
  line L20 (-112.38569, 19.19344) -> (-108.830366, 32.338983)
  arc A41 (-108.830366, 32.338983) -> (-109.14609, 33.360343) centre (-109.795684, 32.600062) ccw
  arc A42 (-110.586613, 35.182536) -> (-109.14609, 33.360343) centre (-105.248527, 37.922031) ccw
  arc A43 (-110.586613, 35.182536) -> (-111.995259, 35.580749) centre (-111.476294, 34.725953) ccw
  line L21 (-111.995259, 35.580749) -> (-127.495344, 26.170308)
  arc A44 (-127.495344, 26.170308) -> (-127.791923, 24.736817) centre (-126.976379, 25.315513) ccw
  arc A45 (-71.858452, 55.325612) -> (-70.160292, 54.741689) centre (-70.866216, 55.449977) ccw
  arc A46 (-69.305274, 55.482332) -> (-70.160292, 54.741689) centre (-64.442314, 49.004554) ccw
  line L22 (-69.305274, 55.482332) -> (-66.550527, 57.55036)
  arc A47 (-66.550527, 57.55036) -> (-66.414464, 59.026602) centre (-67.150892, 58.350086) ccw
  arc A48 (-67.802662, 61.109398) -> (-66.414464, 59.026602) centre (-60.449397, 64.50638) ccw
  arc A49 (-67.802662, 61.109398) -> (-69.229438, 61.544813) centre (-68.710473, 60.690017) ccw
  line L23 (-69.229438, 61.544813) -> (-72.622035, 59.485093)
  arc A50 (-72.622035, 59.485093) -> (-72.918613, 58.051601) centre (-72.10307, 58.630298) ccw
  arc A51 (-71.858452, 55.325612) -> (-72.918613, 58.051601) centre (-77.811872, 54.579424) ccw
  arc A52 (-100.058689, 42.827701) -> (-100.355268, 41.394209) centre (-99.539724, 41.972905) ccw
  arc A53 (-99.420805, 39.349498) -> (-100.355268, 41.394209) centre (-105.248527, 37.922031) ccw
  arc A54 (-99.420805, 39.349498) -> (-98.650829, 38.607882) centre (-98.449518, 39.587409) ccw
  line L24 (-98.650829, 38.607882) -> (-89.908309, 36.81113)
  arc A55 (-89.908309, 36.81113) -> (-88.908264, 37.188973) centre (-89.706998, 37.790657) ccw
  arc A56 (-85.020123, 39.510338) -> (-88.908264, 37.188973) centre (-84.115857, 33.578871) ccw
  arc A57 (-85.020123, 39.510338) -> (-84.213055, 40.211408) centre (-85.170834, 40.498916) ccw
  line L25 (-84.213055, 40.211408) -> (-81.545787, 49.096917)
  arc A58 (-81.545787, 49.096917) -> (-81.833323, 50.126568) centre (-82.503565, 49.384425) ccw
  arc A59 (-83.149958, 51.839928) -> (-81.833323, 50.126568) centre (-77.811872, 54.579424) ccw
  arc A60 (-83.149958, 51.839928) -> (-84.558604, 52.238141) centre (-84.039639, 51.383346) ccw
  line L26 (-84.558604, 52.238141) -> (-100.058689, 42.827701)
  arc A61 (-137.554519, 17.758994) -> (-139.006826, 17.942469) centre (-138.366076, 17.174719) ccw
  line L27 (-139.006826, 17.942469) -> (-143.139417, 14.493481)
  arc A62 (-143.139417, 14.493481) -> (-143.180301, 12.994038) centre (-142.498667, 13.725731) ccw
  arc A63 (-141.858325, 11.317516) -> (-143.180301, 12.994038) centre (-147.951739, 7.872185) ccw
  arc A64 (-141.858325, 11.317516) -> (-140.857998, 10.818171) centre (-140.987838, 11.809706) ccw
  line L28 (-140.857998, 10.818171) -> (-136.934628, 11.331928)
  arc A65 (-136.934628, 11.331928) -> (-136.075602, 12.174654) centre (-137.064468, 12.323463) ccw
  line L29 (-136.075602, 12.174654) -> (-135.604064, 15.308119)
  arc A66 (-135.604064, 15.308119) -> (-136.03468, 16.286601) centre (-136.59293, 15.456928) ccw
  arc A67 (-137.554519, 17.758994) -> (-136.03468, 16.286601) centre (-132.685182, 21.264639) ccw
  arc A68 (-138.19969, 1.899667) -> (-137.500173, 2.708082) centre (-138.489039, 2.856891) ccw
  line L30 (-137.500173, 2.708082) -> (-137.004522, 6.001791)
  arc A69 (-137.004522, 6.001791) -> (-138.123227, 7.142135) centre (-137.993388, 6.1506) ccw
  line L31 (-138.123227, 7.142135) -> (-140.33864, 6.852031)
  arc A70 (-140.33864, 6.852031) -> (-141.176668, 6.111957) centre (-140.2088, 5.860496) ccw
  arc A71 (-144.061428, 2.05278) -> (-141.176668, 6.111957) centre (-147.951739, 7.872185) ccw
  arc A72 (-144.061428, 2.05278) -> (-144.261023, 0.566118) centre (-143.505669, 1.221436) ccw
  line L32 (-144.261023, 0.566118) -> (-143.125657, -0.742563)
  arc A73 (-143.125657, -0.742563) -> (-141.526488, -0.623878) centre (-142.370304, -0.087245) ccw
  arc A74 (-138.19969, 1.899667) -> (-141.526488, -0.623878) centre (-136.463592, -3.843674) ccw
  arc A75 (-76.907606, 48.647957) -> (-74.152214, 49.824752) centre (-77.811872, 54.579424) ccw
  arc A76 (-76.907606, 48.647957) -> (-77.714673, 47.946886) centre (-76.756895, 47.659379) ccw
  line L33 (-77.714673, 47.946886) -> (-80.381942, 39.061377)
  arc A77 (-80.381942, 39.061377) -> (-80.094406, 38.031727) centre (-79.424164, 38.77387) ccw
  arc A78 (-79.072459, 36.829123) -> (-80.094406, 38.031727) centre (-84.115857, 33.578871) ccw
  arc A79 (-79.072459, 36.829123) -> (-77.631528, 36.571106) centre (-78.231893, 37.370832) ccw
  line L34 (-77.631528, 36.571106) -> (-70.457765, 41.956551)
  arc A80 (-70.457765, 41.956551) -> (-70.331118, 43.4429) centre (-71.058131, 42.756277) ccw
  arc A81 (-72.542276, 49.029257) -> (-70.331118, 43.4429) centre (-64.442314, 49.004554) ccw
  arc A82 (-72.542276, 49.029257) -> (-74.152214, 49.824752) centre (-73.542271, 49.032306) ccw
  point P0 (0, 0)
equation "\"d25\" = 0.5 * d24"
equation "\"d46\" = d45"
